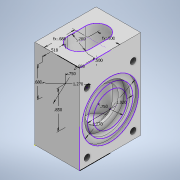
# Autodesk Inventor part: VaporFlowBlock
Saved by Autodesk Inventor 2020 (Build 240168000, 168)
## iProperties
Created: 2020-01-06
Part Number: VaporFlowBlock
Material: Generic
Document SubType Name: Modeling
Designer: pab2
Density: 1 g/cm^3
Appearance: Default
Author: pab2
Autodesk Inventor part; units mm, degrees
ref_plane "YZ Plane" through (0, 0, 0) normal (1, 0, 0) x (0, 1, 0)
ref_plane "XZ Plane" through (0, 0, 0) normal (0, 1, 0) x (-1, 0, 0)
ref_plane "XY Plane" through (0, 0, 0) normal (0, 0, 1) x (1, 0, 0)
sketch "Sketch1" plane through (0, 0, 0) normal (0, 1, 0) x (-1, 0, 0)
  line L0 (0, 0) -> (25.4, 0)
  line L1 (25.4, 0) -> (25.4, -34.925)
  line L2 (25.4, -34.925) -> (0, -34.925)
  line L3 (0, -34.925) -> (0, 0)
  dimension "BlockW" = 25.4
  dimension "BlockL" = 34.925
  constraints: 8 end point, 2 parallel, 1 horizontal, 1 perpendicular
  measures "BlockW" distance of L1.end L2.end
  measures "BlockL" distance of L0.end L1.end
extrude "Extrusion1" add sketch "Sketch1" along normal blind 50.8
sketch "Sketch2" plane through (0, 50.8, 0) normal (0, 1, 0) x (1, 0, 0)
  line L0 (0, 0) -> (-12.7, 0)
  line L1 (0, 17.4625) -> (0, 0)
  line L2 (-12.7, 22.5425) -> (-12.7, 12.3825) construction
  line L3 (-19.05, 22.5425) -> (-19.05, 12.3825)
  line L4 (-6.35, 12.3825) -> (-6.35, 22.5425)
  arc A0 (-6.35, 22.5425) -> (-19.05, 22.5425) centre (-12.7, 22.5425) ccw
  arc A1 (-19.05, 12.3825) -> (-6.35, 12.3825) centre (-12.7, 12.3825) ccw
  line L5 (-12.7, 17.4625) -> (-2.54, 17.4625) construction
  dimension "d4" = 12.7
  dimension "d5" = 17.4625
  dimension "d33" = 5.08
  dimension "d35" = 12.7
  constraints: 14 end point, 4 point on circle, 4 tangent, 2 centre point, 2 horizontal, 1 midpoint, 1 parallel, 1 perpendicular
  measures "d4" distance of L5.start L1.start
  measures "d5" distance of L0.end L5.start
  measures "d33" distance of L5.start L2.end
  measures "d35" diameter of A1
extrude "Extrusion7" cut sketch "Sketch2" against normal blind 44.45
sketch "Sketch3" plane through (0, 0, 0) normal (1, 0, 0) x (0, 0, -1)
  line L0 (0, 0) -> (17.4752, 0)
  line L1 (0, 21.59) -> (0, 0)
  circle A0 centre (17.4752, 21.59) radius 9.525
  circle A1 centre (17.4752, 21.59) radius 12.954
  circle A2 centre (17.4752, 21.59) radius 16.129
  line L2 (4.318, 21.59) -> (21.59, 21.59) construction
  point P0 (4.318, 38.862)
  dimension "d15" = 19.05
  dimension "d16" = 25.908
  dimension "d17" = 32.258
  constraints: 6 end point, 3 centre point, 2 coincident, 2 horizontal
  measures "d15" diameter of A0
  measures "d16" diameter of A1
  measures "d17" diameter of A2
hole "Hole2" at (0, 38.862, -4.318) direction (-1, 0, 0) diameter 3.302 depth 10.16 thread size "8-32 UNC" class "2B" standard "ANSI Unified Screw Threads"
pattern_linear "Rectangular Pattern1" count 2 spacing 26.289 along (0, 0, -1) count 2 spacing 34.544 along (0, -1, 0) of "Hole2"
extrude "Extrusion2" cut sketch "Sketch3" against normal through all contours A0
extrude "Extrusion3" cut sketch "Sketch3" against normal blind 4.826 contours A1
extrude "Extrusion4" cut sketch "Sketch3" against normal blind 1.524 contours A2
sketch "Sketch4" plane through (-25.4, 0, -34.925) normal (-1, 0, 0) x (0, 0, 1)
  line L0 (0, 0) -> (17.4752, 0)
  line L1 (17.4752, 21.59) -> (0, 21.59)
  line L2 (0, 21.59) -> (0, 0)
  circle A0 centre (17.4752, 21.59) radius 9.525
  circle A1 centre (17.4752, 21.59) radius 12.954
  circle A2 centre (17.4752, 21.59) radius 16.129
  line L3 (17.4752, 21.59) -> (30.6197, 21.59)
  line L4 (30.6197, 21.59) -> (30.6197, 38.862)
  line L5 (30.6197, 38.862) -> (17.4752, 38.862)
  line L6 (17.4752, 38.862) -> (17.4752, 21.59)
  point P0 (34.925, 0)
  dimension "d24" = 17.4752
  dimension "d25" = 21.59
  dimension "d26" = 19.05
  dimension "d28" = 32.258
  dimension "d57" = 13.1445
  dimension "d58" = 17.272
  constraints: 14 end point, 3 centre point, 3 coincident, 3 parallel, 2 horizontal, 1 perpendicular
  measures "d24" distance of L1.end L1.start
  measures "d25" distance of L1.start L0.end
  measures "d26" diameter of A0
  measures "d28" diameter of A2
  measures "d57" distance of L5.end L4.end
  measures "d58" distance of L4.end L3.end
extrude "Extrusion5" cut sketch "Sketch4" against normal blind 4.826 contours A0 L3 A1 L1 | L1 A1 L6 A0 | A0 L6 A1 L3
extrude "Extrusion6" cut sketch "Sketch4" against normal blind 1.524 contours A1 L3 L4 A2 L1 | L1 A2 L6 A1 | A1 L6 A2 L4 L3
hole "Hole3" at (-25.4, 38.862, -4.3053) direction (1, 0, 0) diameter 3.302 depth 10.16 thread size "8-32 UNC" class "2B" standard "ANSI Unified Screw Threads"
pattern_linear "Rectangular Pattern2" count 2 spacing 26.289 along (0, 0, -1) count 2 spacing 34.544 along (0, -1, 0) of "Hole3"
equation "\"d4\" = 0.5 * BlockW"
equation "\"d5\" = 0.5 * BlockL"
equation "\"d36\" = WellDepth"
equation "\"WellDepth\" = 44.45"
body "Solid1"
